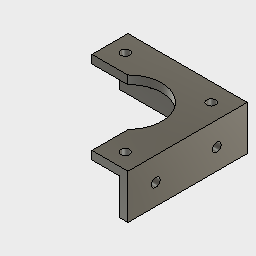
XYMotorMount (Autodesk Fusion 360 design; units mm, degrees)
Autodesk Fusion 360 part; units mm, degrees
sketch "Sketch1" plane through (0, 0, 0) normal (0, 0, 1) x (1, 0, 0) in component "Component"
  line L0 (0, 0) -> (-43, 0)
  line L1 (-43, 0) -> (-43, -43)
  line L2 (-43, -43) -> (0, -43)
  line L3 (0, -43) -> (0, 0)
  dimension "d1" = 43
  dimension "d2" = 43
  constraint horizontal L0
  constraint vertical L1
  constraint horizontal L2
  constraint vertical L3
extrude "Extrude1" add sketch "Sketch1" along normal blind 16 in component "Component"
sketch "Sketch2" plane through (0, 0, 0) normal (0, 0, -1) x (1, 0, 0) in component "Component"
  line L0 (0, 0) -> (0, 43)
  line L1 (0, 43) -> (-43, 43)
  line L2 (-43, 43) -> (-43, 0)
  line L3 (-43, 0) -> (0, 0)
  line L4 (-43, 43) -> (-3, 43)
  line L5 (-3, 43) -> (-3, 3)
  line L6 (-3, 3) -> (-43, 3)
  line L7 (-43, 3) -> (-43, 43)
  dimension "d5" = 40
  dimension "d6" = 40
  constraint horizontal L4
  constraint vertical L5
  constraint horizontal L6
  constraint vertical L7
extrude "Extrude2" cut sketch "Sketch2" against normal blind 13 contours L1 L2 L4 L5 L6 L7 in component "Component"
sketch "Sketch3" plane through (0, 0, 16) normal (0, 0, 1) x (-1, 0, 0) in component "Component"
  line L0 (0, 43) -> (0, 0)
  line L1 (0, 0) -> (43, 0)
  line L2 (43, 0) -> (43, 43)
  line L3 (43, 43) -> (0, 43)
  line L4 (43, 43) -> (13, 43)
  line L5 (13, 43) -> (13, 13)
  line L6 (13, 13) -> (43, 13)
  line L7 (43, 13) -> (43, 43)
  dimension "d9" = 30
  dimension "d10" = 30
  constraint horizontal L4
  constraint vertical L5
  constraint horizontal L6
  constraint vertical L7
extrude "Extrude3" cut sketch "Sketch3" against normal up to surface (3 mm away) contours L2 L3 L4 L5 L6 L7 in component "Component"
sketch "Sketch4" plane through (0, 0, 16) normal (0, 0, 1) x (-1, 0, 0) in component "Component"
  line L0 (13, 13) -> (13, 43)
  line L1 (13, 43) -> (0, 43)
  line L2 (0, 43) -> (0, 0)
  line L3 (0, 0) -> (43, 0)
  line L4 (43, 0) -> (43, 13)
  line L5 (43, 13) -> (13, 13)
  line L6 (13, 43) -> (13, 29.6854)
  line L7 (13, 43) -> (26, 43) construction
  line L8 (43, 13) -> (30, 13)
  line L9 (43, 13) -> (56, 13) construction
  line L10 (13, 29.6854) -> (30, 13) construction
  line L11 (13, 13) -> (27.8599, 28.1401) construction
  circle A0 centre (21.5, 21.3427) radius 12
  line L12 (30, 13) -> (30.1255, 13)
  line L13 (13, 29.6854) -> (13, 29.8133)
  dimension "d12" = 90
  dimension "d14" = 180
  dimension "d16" = 24
  constraint horizontal L7
  constraint horizontal L9
  constraint perpendicular L10 L11
  constraint midpoint L10
  constraint coincident A0
  constraint coincident L5
  constraint coincident L0
  measures "d12" angle of L6 L7
  measures "d14" angle of L8 L9
  measures "d16" diameter of A0
extrude "Extrude4" cut sketch "Sketch4" against normal up to surface (3 mm away) contours L0 L5 L6 L8 A0 L12 L13 | L0 L5 L6 L8 A0 L12 L13 in component "Component"
sketch "Sketch5" plane through (0, 0, 16) normal (0, 0, 1) x (-1, 0, 0) in component "Component"
  arc A0 (13, 29.8133) -> (30.1255, 13) centre (21.5, 21.3427) ccw
  line L0 (13, 29.8133) -> (13, 43)
  line L1 (13, 43) -> (0, 43)
  line L2 (0, 43) -> (0, 0)
  line L3 (0, 0) -> (43, 0)
  line L4 (43, 0) -> (43, 13)
  line L5 (43, 13) -> (30.1255, 13)
  circle A1 centre (37.5, 6.5) radius 1.6
  circle A2 centre (6.5, 6.5) radius 1.6
  circle A3 centre (6.5, 37.5) radius 1.6
  dimension "d18" = 3.2
  dimension "d19" = 3.2
  dimension "d20" = 3.2
  dimension "d25" = 5.5
  dimension "d26" = 6.5
  dimension "d27" = 6.5
  dimension "d28" = 5.5
  dimension "d29" = 6.5
  dimension "d30" = 6.5
  measures "d18" diameter of A1
  measures "d19" diameter of A2
  measures "d20" diameter of A3
  measures "d25" distance of L4
  measures "d26" distance of L3
  measures "d27" distance of L2
  measures "d28" distance of L1
  measures "d29" distance of L3
  measures "d30" distance of L2
sketch "Sketch6" plane through (0, 0, 0) normal (0, 1, 0) x (-1, 0, 0) in component "Component"
  line L0 (0, 0) -> (43, 0)
  line L1 (43, 0) -> (43, 16)
  line L2 (43, 16) -> (0, 16)
  line L3 (0, 16) -> (0, 0)
  circle A0 centre (32, 7.5) radius 1.6
  circle A1 centre (10, 7.5) radius 1.6
  dimension "d21" = 3.2
  dimension "d22" = 3.2
  dimension "d32" = 8.5
  dimension "d33" = 8.5
  dimension "d34" = 10
  dimension "d35" = 11
  measures "d21" diameter of A0
  measures "d22" diameter of A1
  measures "d32" distance of L2
  measures "d33" distance of L2
  measures "d34" distance of L3
  measures "d35" distance of L1
sketch "Sketch7" plane through (0, 0, 0) normal (1, 0, 0) x (0, 1, 0) in component "Component"
  line L0 (-43, 0) -> (0, 0)
  line L1 (0, 0) -> (0, 16)
  line L2 (0, 16) -> (-43, 16)
  line L3 (-43, 16) -> (-43, 0)
  circle A0 centre (-11, 7.5) radius 1.6
  circle A1 centre (-33, 7.5) radius 1.6
  dimension "d23" = 3.2
  dimension "d24" = 3.2
  dimension "d37" = 8.5
  dimension "d38" = 8.5
  dimension "d39" = 11
  dimension "d40" = 10
  dimension "d41" = 22
  constraint midpoint L1
  constraint midpoint L3
  measures "d23" diameter of A0
  measures "d24" diameter of A1
  measures "d37" distance of L2
  measures "d38" distance of L2
extrude "Extrude5" cut sketch "Sketch5" against normal up to surface (3 mm away) contours A1 | A2 | A3 in component "Component"
extrude "Extrude6" cut sketch "Sketch6" against normal up to surface (3 mm away) contours A0 | A1 in component "Component"
extrude "Extrude7" cut sketch "Sketch7" against normal up to surface (3 mm away) contours A0 | A1 in component "Component"
component "Component" placed x (1, 0, 0) y (0, 1, 0) z (0, 0, 1) at (0, 0, 0)
equation "d33 = d32"
equation "d37 = d32"
equation "d38 = d32"
